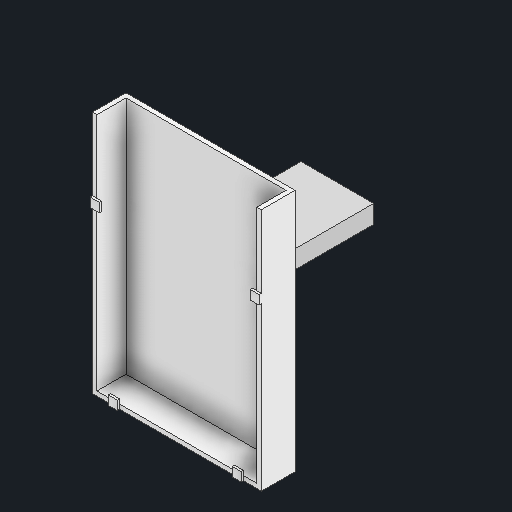
# Autodesk Inventor part: MovingCompartment
Saved by Autodesk Inventor 2025 (Build 290162000, 162)
## iProperties
Created: 2024-04-22
Part Number: MovingCompartment
Material: Generic
Document SubType Name: Modeling
Designer: conno
Density: 1 g/cm^3
Appearance: Default
Author: conno
Autodesk Inventor part; units mm, degrees
ref_plane "YZ Plane" through (0, 0, 0) normal (1, 0, 0) x (0, 1, 0)
ref_plane "XZ Plane" through (0, 0, 0) normal (0, 1, 0) x (-1, 0, 0)
ref_plane "XY Plane" through (0, 0, 0) normal (0, 0, 1) x (1, 0, 0)
sketch "Sketch1" plane through (0, 0, 0) normal (0, 0, 1) x (1, 0, 0)
  line L0 (28.0448, -41.9322) -> (-28.0448, -41.9322)
  line L1 (-28.0448, -41.9322) -> (-28.0448, 41.9322)
  line L2 (-28.0448, 41.9322) -> (28.0448, 41.9322)
  line L3 (28.0448, 41.9322) -> (28.0448, -41.9322)
  line L4 (28.0448, -41.9322) -> (-28.0448, 41.9322) construction
  line L5 (-28.0448, -41.9322) -> (28.0448, 41.9322) construction
  point P0 (0, 0)
  dimension "d0" = 56.0896
  dimension "d1" = 83.8645
  constraints: 12 end point, 2 midpoint, 2 parallel, 1 horizontal, 1 perpendicular
  measures "d0" distance of L1.end L2.end
  measures "d1" distance of L0.end L1.end
extrude "Container Backplate" add sketch "Sketch1" along normal mid plane 1.5875
sketch "Sketch2" plane through (0, 0, -0.7937) normal (0, 0, -1) x (-1, 0, 0)
  line L0 (28.0448, 41.9322) -> (-28.0448, 41.9322) projected
  line L1 (-28.0448, 41.9322) -> (-28.0448, -41.9322) projected
  line L2 (-28.0448, -41.9322) -> (28.0448, -41.9322) projected
  line L3 (28.0448, -41.9322) -> (28.0448, 41.9322) projected
  line L4 (-29.6323, 43.5197) -> (29.6323, 43.5197)
  line L5 (29.6323, 43.5197) -> (29.6323, -43.5197)
  line L6 (29.6323, -43.5197) -> (-29.6323, -43.5197)
  line L7 (-29.6323, -43.5197) -> (-29.6323, 43.5197)
  line L8 (28.0448, 41.9322) -> (29.6323, 41.9322)
  line L9 (-28.0448, 41.9322) -> (-29.6323, 41.9322)
  point P0 (0, 0)
  point P1 (28.0448, 43.5197)
  point P2 (-28.0448, 43.5197)
  dimension "d4" = 1.5875
  constraints: 12 end point, 4 point on line, 1 horizontal, 1 perpendicular, 3 other
  measures "d4" distance between parallel lines of L0 L4
extrude "Container Walls" add sketch "Sketch2" against normal blind 11.7792 contours L8 L5 L6 L7 L9 L1 L2 L3
sketch "Sketch3" plane through (0, 0, 10.9855) normal (0, 0, 1) x (1, 0, 0)
  line L0 (-23.2823, -43.5197) -> (-20.1073, -43.5197)
  line L1 (-20.1073, -43.5197) -> (-20.1073, -40.3447)
  line L2 (-20.1073, -40.3447) -> (-23.2823, -40.3447)
  line L3 (-23.2823, -40.3447) -> (-23.2823, -43.5197)
  line L4 (-29.6323, -43.5197) -> (29.6323, -43.5197) projected
  line L5 (28.0448, -41.9322) -> (-28.0448, -41.9322) projected
  line L6 (-29.6323, 41.9322) -> (-29.6323, -43.5197) projected
  line L7 (-29.6323, 16.5322) -> (-26.4573, 16.5322)
  line L8 (-26.4573, 16.5322) -> (-26.4573, 13.3572)
  line L9 (-26.4573, 13.3572) -> (-29.6323, 13.3572)
  line L10 (-29.6323, 13.3572) -> (-29.6323, 16.5322)
  line L11 (28.0448, 41.9322) -> (-28.0448, 41.9322) projected
  line L12 (0, 41.9322) -> (0, -43.5197)
  line L13 (23.2823, -43.5197) -> (20.1073, -43.5197)
  line L14 (20.1073, -43.5197) -> (20.1073, -40.3447)
  line L15 (20.1073, -40.3447) -> (23.2823, -40.3447)
  line L16 (23.2823, -40.3447) -> (23.2823, -43.5197)
  line L17 (29.6323, 43.5197) -> (29.6323, -43.5197)
  line L18 (29.6323, 16.5322) -> (26.4573, 16.5322)
  line L19 (26.4573, 16.5322) -> (26.4573, 13.3572)
  line L20 (26.4573, 13.3572) -> (29.6323, 13.3572)
  line L21 (29.6323, 13.3572) -> (29.6323, 16.5322)
  point P0 (0, 0)
  point P1 (-29.6323, 43.5197)
  dimension "d7" = 3.175
  dimension "d8" = 3.175
  dimension "d9" = 6.35
  dimension "d10" = 3.175
  dimension "d11" = 3.175
  dimension "d12" = 25.4
  constraints: 36 end point, 9 symmetric about line, 4 parallel, 2 horizontal, 2 midpoint, 2 perpendicular, 2 point on line, 1 collinear
  measures "d7" distance of L2.end L1.end
  measures "d8" distance of L1.end L0.end
  measures "d9" distance between parallel lines of L6 L3
  measures "d10" distance of L8.end L9.end
  measures "d11" distance of L7.end L8.end
  measures "d12" distance between parallel lines of L11 L7
extrude "Container Tabs" add sketch "Sketch3" along normal blind 0.7937 contours L3 L5 L1 L0 | L20 L19 L18 L17 | L6 L7 L8 L9 | L3 L2 L1 L5 | L14 L5 L16 L4 | L14 L15 L16 L5
sketch "Sketch11" plane through (0, 0, -0.7937) normal (0, 0, -1) x (-1, 0, 0)
  line L0 (-12.7381, 7.2803) -> (12.7381, 7.2803)
  line L1 (12.7381, 7.2803) -> (12.7381, 0.9303)
  line L2 (12.7381, 0.9303) -> (-12.7381, 0.9303)
  line L3 (-12.7381, 0.9303) -> (-12.7381, 7.2803)
  line L4 (-29.6323, -43.5197) -> (29.6323, -43.5197) projected
  point P0 (0, 0)
  point P1 (0, 7.2803)
  dimension "d58" = 25.4762
  dimension "d59" = 6.35
  dimension "d60" = 44.45
  constraints: 8 end point, 2 parallel, 1 horizontal, 1 midpoint, 1 perpendicular, 1 vertical alignment
  measures "d58" distance of L1.end L2.end
  measures "d59" distance of L0.end L1.end
  measures "d60" distance between parallel lines of L4 L2
extrude "Servo Connector Tab" add sketch "Sketch11" along normal blind 44.45
body "Solid1"
